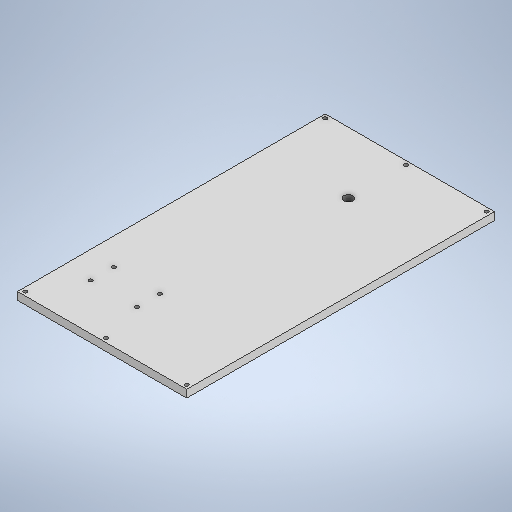
# Autodesk Inventor part: chassis_haut
Saved by Autodesk Inventor 2026.2 (Build 302298010, 298A)
## iProperties
Created: 2026-03-16
Part Number: chassis_haut
Material: Générique
Document SubType Name: Modeling
Designer: genon
Density: 1 g/cm^3
Appearance: Par défaut
Author: genon
Autodesk Inventor part; units mm, degrees
ref_plane "YZ Plane" through (0, 0, 0) normal (1, 0, 0) x (0, 1, 0)
ref_plane "XZ Plane" through (0, 0, 0) normal (0, 1, 0) x (-1, 0, 0)
ref_plane "XY Plane" through (0, 0, 0) normal (0, 0, 1) x (1, 0, 0)
sketch "Esquisse1" plane through (0, 0, 0) normal (0, 1, 0) x (-1, 0, 0)
  line L0 (-55, 100) -> (55, 100)
  line L1 (55, 100) -> (55, -100)
  line L2 (55, -100) -> (-55, -100)
  line L3 (-55, -100) -> (-55, 100)
  line L4 (-55, 100) -> (55, -100) construction
  line L5 (55, 100) -> (-55, -100) construction
  point P0 (0, 0)
  dimension "d0" = 110
  dimension "d1" = 200
  constraints: 12 end point, 2 midpoint, 2 parallel, 1 horizontal, 1 perpendicular
  measures "d0" distance of L1.end L2.end
  measures "d1" distance of L0.end L1.end
extrude "Extrusion1" add sketch "Esquisse1" along normal blind 5
sketch "Esquisse2" plane through (0, 5, 0) normal (0, 1, 0) x (1, 0, 0)
  line L0 (0, 0) -> (0, -97.5)
  line L1 (0, -97.5) -> (-52.5, -97.5)
  line L2 (0, 0) -> (-32.0024, 0)
  point P0 (52.5, -97.5)
  point P1 (-52.5, 97.5)
  point P2 (52.5, 97.5)
  dimension "d4" = 97.5
  dimension "d5" = 52.5
  constraints: 6 end point, 3 symmetric about line, 1 coincident, 1 horizontal, 1 perpendicular, 1 vertical
  measures "d4" distance of L0.start L0.end
  measures "d5" distance of L0.end L1.end
hole "Perçage1" at (-52.5, 5, 97.5) at (52.5, 5, 97.5) at (-52.5, 5, -97.5) at (52.5, 5, -97.5) direction (0, -1, 0) diameter 2.459 end through all thread size "M3x0.5" class "6H" standard "ISO Metric profile"
sketch "Esquisse3" plane through (0, 5, 0) normal (0, 1, 0) x (1, 0, 0)
  line L0 (0, 0) -> (-87.5, 0)
  line L1 (0, 0) -> (0, 97.5)
  point P0 (87.5, 0)
  point P1 (0, -97.5)
  dimension "d13" = 87.5
  dimension "d14" = 97.5
  constraints: 4 end point, 2 coincident, 2 symmetric about line, 1 horizontal, 1 vertical
  measures "d13" distance of L0.start L0.end
  measures "d14" distance of L0.start L1.end
hole "Perçage2" at (-87.5, 5, 0) at (0, 5, -97.5) at (87.5, 5, 0) at (0, 5, 97.5) direction (0, -1, 0) diameter 2.459 end through all thread size "M3x0.5" class "6H" standard "ISO Metric profile"
sketch "Esquisse4" plane through (0, 5, 0) normal (0, 1, 0) x (1, 0, 0)
  line L0 (0, 0) -> (0, 60)
  dimension "d22" = 60
  constraints: 2 end point, 1 coincident, 1 vertical
  measures "d22" distance of L0.start L0.end
hole "Perçage3" at (0, 5, -60) direction (0, -1, 0) diameter 5.9175 end through all thread size "M7x1" class "6H" standard "ISO Metric profile"
sketch "Esquisse5" plane through (0, 5, 0) normal (0, 1, 0) x (1, 0, 0)
  line L0 (-55, -100) -> (55, -100) projected
  line L1 (0, -100) -> (-27.5, -100)
  line L2 (-27.5, -100) -> (-27.5, -70)
  line L3 (-27.5, -70) -> (-37.5, -70)
  line L4 (-27.5, -70) -> (-7.5, -70)
  line L5 (-37.5, -70) -> (-37.5, -55)
  line L6 (-7.5, -55) -> (-7.5, -70)
  point P0 (0, 0)
  dimension "d30" = 27.5
  dimension "d31" = 30
  dimension "d32" = 10
  dimension "d33" = 20
  dimension "d34" = 15
  constraints: 12 end point, 4 coincident, 2 horizontal, 2 vertical, 1 midpoint, 1 perpendicular, 1 point on line
  measures "d30" distance of L1.start L1.end
  measures "d31" distance of L1.end L2.end
  measures "d32" distance of L2.end L3.end
  measures "d33" distance of L2.end L4.end
  measures "d34" distance of L5.start L5.end
hole "Perçage4" at (-7.5, 5, 70) at (-37.5, 5, 70) at (-37.5, 5, 55) at (-7.5, 5, 55) direction (0, -1, 0) diameter 2.459 end through all thread size "M3x0.5" class "6H" standard "ISO Metric profile"
